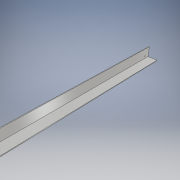
# Autodesk Inventor part: Profile-L-30x30x2
Saved by Autodesk Inventor 2018 (Build 220112000, 112)
## iProperties
Created: 2025-02-16
Part Number: Profile-L-30x30x2
Material: Všeobecné
Document SubType Name: Modeling
Designer: Jozko Mrkvicka
Density: 1 g/cm^3
Appearance: Výchozí
Author: Jozko Mrkvicka
Autodesk Inventor part; units mm, degrees
ref_plane "YZ Plane" through (0, 0, 0) normal (1, 0, 0) x (0, 1, 0)
ref_plane "XZ Plane" through (0, 0, 0) normal (0, 1, 0) x (-1, 0, 0)
ref_plane "XY Plane" through (0, 0, 0) normal (0, 0, 1) x (1, 0, 0)
sketch "Náčrt1" plane through (0, 0, 0) normal (0, 0, 1) x (1, 0, 0)
  line L0 (0, 0) -> (30, 0)
  line L1 (30, 0) -> (30, 2)
  line L2 (30, 2) -> (2, 2)
  line L3 (2, 2) -> (2, 30)
  line L4 (2, 30) -> (0, 30)
  line L5 (0, 30) -> (0, 0)
  dimension "d11" = 30
  dimension "d12" = 30
  dimension "d13" = 2
  dimension "d14" = 2
  constraints: 12 end point, 3 perpendicular, 2 vertical, 1 horizontal
  measures "d11" distance of L0.start L0.end
  measures "d12" distance of L4.end L0.start
  measures "d13" distance of L3.end L4.end
  measures "d14" distance of L0.end L1.end
extrude "Vysunutí1" add sketch "Náčrt1" along normal blind 460
sketch "Náčrt2" plane through (2, 2, 0) normal (0, 1, 0) x (1, 0, 0)
  line L0 (0, 0) -> (0, -460) projected
  line L1 (28, -460) -> (0, -460) projected
  circle A0 centre (7, -445) radius 1.5
  line L2 (28, 0) -> (28, -460) projected
  line L3 (28, -230) -> (0, -230)
  circle A1 centre (7, -15) radius 1.5
  point P0 (-2, 0)
  dimension "d7" = 15
  dimension "d8" = 3
  constraints: 2 centre point, 2 end point, 2 midpoint, 1 symmetric about line, 1 other
  measures "d7" distance from line of A0.centre L1
  measures "d8" diameter of A0
extrude "Vysunutí2" cut sketch "Náčrt2" against normal up to next contours A0 | A1
